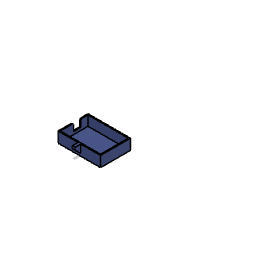
Tiroir (Autodesk Fusion 360 design; units mm, degrees)
Autodesk Fusion 360 part; units mm, degrees
note: some values were not read from the file. Set by a fixed rule: which sketch regions a step uses.
sketch "Sketch1" plane through (0, 3, 0) normal (0, 1, 0) x (-1, 0, 0)
  line L0 (-66.9136, -30.1089) -> (-66.9136, -18.8089)
  line L1 (-66.9136, -18.8089) -> (-57.9136, -18.8089)
  line L2 (-57.9136, -18.8089) -> (-57.9136, -30.1089)
  line L3 (-57.9136, -30.1089) -> (-66.9136, -30.1089)
  line L4 (28.0864, 127.4911) -> (37.0864, 127.4911)
  line L5 (37.0864, 127.4911) -> (37.0864, 116.1911)
  line L6 (37.0864, 116.1911) -> (28.0864, 116.1911)
  line L7 (28.0864, 116.1911) -> (28.0864, 127.4911)
  circle A0 centre (-47.9136, 29.4911) radius 5.65
  circle A1 centre (-47.9136, -23.8089) radius 5.65
  circle A2 centre (18.0864, -23.8089) radius 5.65
  circle A3 centre (18.0864, 29.4911) radius 5.65
  line L8 (39.0864, 128.1911) -> (-68.9136, 128.1911)
  line L9 (-68.9136, 128.1911) -> (-68.9136, -30.8089)
  line L10 (-68.9136, -30.8089) -> (39.0864, -30.8089)
  line L11 (39.0864, -30.8089) -> (39.0864, 128.1911)
  line L12 (37.0864, -30.1089) -> (28.0864, -30.1089)
  line L13 (28.0864, -30.1089) -> (28.0864, -18.8089)
  line L14 (28.0864, -18.8089) -> (37.0864, -18.8089)
  line L15 (37.0864, -18.8089) -> (37.0864, -30.1089)
  line L16 (-57.9136, 127.4911) -> (-57.9136, 116.1911)
  line L17 (-57.9136, 116.1911) -> (-66.9136, 116.1911)
  line L18 (-66.9136, 116.1911) -> (-66.9136, 127.4911)
  line L19 (-66.9136, 127.4911) -> (-57.9136, 127.4911)
  line L20 (24.0864, 76.1911) -> (-53.9136, 76.1911)
  line L21 (-53.9136, 76.1911) -> (-53.9136, 131.1911)
  line L22 (-53.9136, 131.1911) -> (24.0864, 131.1911)
  line L23 (24.0864, 131.1911) -> (24.0864, 76.1911)
  line L24 (-51.9136, 129.1911) -> (22.0864, 129.1911)
  line L25 (22.0864, 129.1911) -> (22.0864, 78.1911)
  line L26 (22.0864, 78.1911) -> (-51.9136, 78.1911)
  line L27 (-51.9136, 78.1911) -> (-51.9136, 129.1911)
  dimension "d289" = 78
  dimension "d290" = 55
  dimension "d293" = 2
  dimension "d294" = 15
  dimension "d295" = 3
  constraint horizontal L20
  constraint vertical L21
  constraint horizontal L22
  constraint vertical L23
  measures "d289" distance of L20.start L20.end
  measures "d290" distance of L20.start L22.end
  measures "d294" distance of L9 L21
  measures "d295" distance of L8 L22
extrude "Extrude1" add sketch "Sketch1" along normal blind 20 contours L8 L20 L21 L23 L25 L26 L27 | L8 L21 L22 L23 L24 L25 L27
extrude "Extrude2" add sketch "Sketch1" along normal blind 2 contours L8 L25 L26 L27 | L8 L24 L25 L27
sketch "Sketch2" plane through (-22.0864, 0, 0) normal (1, 0, 0) x (0, 0, -1)
  line L0 (-129.1911, 5) -> (-78.1911, 5)
  line L1 (-78.1911, 5) -> (-78.1911, 23)
  line L2 (-78.1911, 23) -> (-129.1911, 23)
  line L3 (-129.1911, 23) -> (-129.1911, 5)
  line L4 (-104.6174, 23) -> (-91.4422, 23)
  line L5 (-91.4422, 23) -> (-91.4422, 9.845)
  line L6 (-91.4422, 9.845) -> (-104.6174, 9.845)
  line L7 (-104.6174, 9.845) -> (-104.6174, 23)
  constraint horizontal L4
  constraint vertical L5
  constraint horizontal L6
  constraint vertical L7
  constraint coincident L2 L4.start
extrude "Extrude3" cut sketch "Sketch2" against normal blind 2 contours L2 L4 L5 L6 L7
ref_plane "WorkPlane1" through (17.4136, 13, 103.6911) normal (1, 0, 0) x (0, 0, -1)
sketch "Bouton" plane through (17.4136, 13, 103.6911) normal (1, 0, 0) x (0, 0, -1)
  line L0 (-37.5, 10) -> (-27.5, 10)
  line L1 (-27.5, 10) -> (27.5, 10)
  line L2 (-27.5, -10) -> (-27.5, 10)
  line L3 (-37.5, 10) -> (-24.3614, 10) construction
  line L4 (-37.5, 5) -> (-27.5, -5)
  line L5 (-37.5, 5) -> (-29.1688, 5) construction
  spline S0 degree 5 poles (-37.5, 5) (-37.5776, 5.1802) (-37.7238, 5.5429) (-37.9161, 6.0939) (-38.1146, 6.8433) (-38.219, 7.8167) (-38.1152, 8.6431) (-37.879, 9.3034) (-37.64, 9.7643) (-37.5, 10) knots 0 0 0 0 0 0 0.2 0.4 0.6 0.8 1 1 1 1 1 1
  line L6 (-37.8335, 9.4384) -> (-37.1665, 10.5616)
  dimension "d349" = 10
  dimension "d353" = 5
  dimension "d354" = 45
  constraint horizontal L0
  constraint coincident L0.end L1.start
  constraint horizontal L3
  constraint horizontal L5
  constraint coincident L2 L4.end
  constraint midpoint L0.start L6
  measures "d349" distance of L0.start L0.end
  measures "d353" distance of L0.start L4.start
  measures "d354" angle of L4 L5
extrude "Extrude4" add sketch "Bouton" against normal blind 5
chamfer "Chamfer1" distance 0.6 angle 45 4 edges at (53.9136, 3, 103.6911) (14.9136, 3, 131.1911) (-24.0864, 3, 103.6911) (14.9136, 3, 76.1911)
chamfer "Chamfer3" distance 2 angle 45 2 edges at (-23.0864, 23, 91.4422) (-23.0864, 23, 104.6174)
equation "d289 = LargeurTiroir"
equation "d290 = ProfondeurTiroir"
equation "d294 = ( Largeur - LargeurTiroir ) / 2"
equation "d295 = EpaisseurParoi"
equation "d348 = -LargeurTiroir / 2 + LargeurBouton / 2"
equation "d355 = -LargeurBouton"
equation "Largeur = 108 mm"
equation "EpaisseurParoi = 3 mm"
equation "ProfondeurTiroir = 55 mm"
equation "LargeurTiroir = 78 mm"
equation "LargeurBouton = 5 mm"
